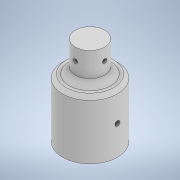
# Autodesk Inventor part: shaft adapter
Saved by Autodesk Inventor 2020.3 (Build 243373000, 373)
## iProperties
Created: 2020-09-03
Part Number: shaft adapter
Material: Generic
Document SubType Name: Modeling
Designer: joesp
Density: 1 g/cm^3
Appearance: Default
Author: joesp
Autodesk Inventor part; units mm, degrees
ref_plane "YZ Plane" through (0, 0, 0) normal (1, 0, 0) x (0, 1, 0)
ref_plane "XZ Plane" through (0, 0, 0) normal (0, 1, 0) x (-1, 0, 0)
ref_plane "XY Plane" through (0, 0, 0) normal (0, 0, 1) x (1, 0, 0)
sketch "Sketch1" plane through (0, 0, 0) normal (0, 1, 0) x (-1, 0, 0)
  circle A0 centre (0, 0) radius 12
  circle A1 centre (0, 0) radius 22.5
  line L0 (11.619, 3) -> (16.619, 3)
  line L1 (16.619, 3) -> (16.619, -3)
  line L2 (16.619, -3) -> (11.619, -3)
  line L3 (11.619, -3) -> (11.619, 3)
  dimension "d0" = 24
  dimension "d1" = 45
  dimension "d2" = 6
  dimension "d3" = 5
  constraints: 8 end point, 2 centre point, 2 coincident, 2 parallel, 2 point on circle, 1 horizontal, 1 perpendicular
  measures "d0" diameter of A0
  measures "d1" diameter of A1
  measures "d2" distance of L0.end L1.end
  measures "d3" distance of L0.start L0.end
extrude "Extrusion1" add sketch "Sketch1" along normal blind 40
sketch "Sketch2" plane through (0, 40, 0) normal (0, 1, 0) x (1, 0, 0)
  circle A0 centre (0, 0) radius 22.5
  constraints: 1 centre point, 1 coincident
extrude "Extrusion2" add sketch "Sketch2" along normal blind 8
sketch "Sketch3" plane through (0, 48, 0) normal (0, 1, 0) x (1, 0, 0)
  circle A0 centre (0, 0) radius 12
  dimension "d29" = 24
  constraints: 1 centre point, 1 coincident
  measures "d29" diameter of A0
extrude "Extrusion3" add sketch "Sketch3" along normal blind 25
sketch "Sketch4" plane through (0, 0, 0) normal (1, 0, 0) x (0, 1, 0)
  circle A0 centre (63, 0) radius 1.75
  line L0 (48, -22.5) -> (48, 22.5) projected
  point P0 (0, 0)
  dimension "d10" = 15
  dimension "d11" = 3.5
  constraints: 1 centre point
  measures "d10" distance from line of L0 A0.centre
  measures "d11" diameter of A0
extrude "Extrusion4" cut sketch "Sketch4" along normal through all both and the other way through all
sketch "Sketch5" plane through (0, 0, 0) normal (0, 0, 1) x (1, 0, 0)
  circle A0 centre (0, 63) radius 1.75
  line L0 (-12, 64.75) -> (12, 64.75) projected
  line L1 (22.5, 48) -> (-22.5, 48) projected
  point P0 (0, 0)
  dimension "d14" = 15
  constraints: 1 centre point, 1 tangent
  measures "d14" distance from line of L1 A0.centre
extrude "Extrusion5" cut sketch "Sketch5" along normal through all both and the other way through all
sketch "Sketch6" plane through (0, 0, 0) normal (1, 0, 0) x (0, 1, 0)
  circle A0 centre (24, 0) radius 2
  line L0 (0, -22.5) -> (0, 22.5) projected
  line L1 (48, -22.5) -> (48, 22.5) projected
  point P0 (0, 0)
  dimension "d18" = 4
  dimension "d19" = 24
  dimension "d20" = 24
  constraints: 1 centre point, 1 horizontal alignment
  measures "d18" diameter of A0
  measures "d19" distance from line of L0 A0.centre
  measures "d20" distance from line of L1 A0.centre
extrude "Extrusion6" cut sketch "Sketch6" along normal through all
chamfer "Chamfer1" distance 3 angle 45 1 edges at (-22.5, 48, 0)
chamfer "Chamfer2" distance 5 angle 45 1 edges at (-12, 48, 0)
equation "\"d19\" = d20"
body "Solid1"
